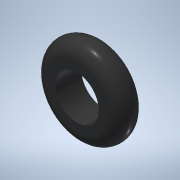
# Autodesk Inventor part: shocks_rubber
Saved by Autodesk Inventor 2020 (Build 240168000, 168)
## iProperties
Created: 2015-12-02
Part Number: shocks_rubber
Material: Goma
Document SubType Name: Modeling
Designer: MIGUEL ANGEL
Density: 0.93 g/cm^3
Appearance: Goma - Negro - Versión 1.1
Author: MIGUEL ANGEL
Autodesk Inventor part; units mm, degrees
ref_plane "YZ Plane" through (0, 0, 0) normal (1, 0, 0) x (0, 1, 0)
ref_plane "XZ Plane" through (0, 0, 0) normal (0, 1, 0) x (-1, 0, 0)
ref_plane "XY Plane" through (0, 0, 0) normal (0, 0, 1) x (1, 0, 0)
sketch "Boceto1" plane through (0, 0, 0) normal (0, 1, 0) x (-1, 0, 0)
  circle A0 centre (0, 0) radius 5
  dimension "d0" = 10
  constraints: 1 centre point, 1 coincident
  measures "d0" diameter of A0
extrude "Extrusión1" add sketch "Boceto1" along normal blind 3
sketch "Boceto2" plane through (0, 3, 0) normal (0, 1, 0) x (1, 0, 0)
  circle A0 centre (0, 0) radius 2.5
  dimension "d3" = 5
  constraints: 1 centre point, 1 coincident
  measures "d3" diameter of A0
extrude "Extrusión2" cut sketch "Boceto2" against normal through all
fillet "Empalme1" radius 1.5 2 edges at (5, 3, 0) (5, 0, 0)
